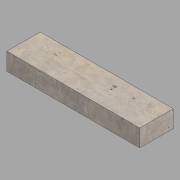
# Autodesk Inventor part: Paver type 2-pedestrian
Saved by Autodesk Inventor 2022 (Build 260153000, 153)
## iProperties
Created: 2021-10-21
Part Number: Paver type 2-pedestrian
Material: Limestone
Document SubType Name: Modeling
Designer: awelt
Density: 2.6 g/cm^3
Appearance: Kasota Gray
Mass: 19098 g
Surface Area: 3056.7 cm^2
Volume: 7345.37 cm^3
Author: awelt
Autodesk Inventor part; units mm, degrees
ref_plane "YZ Plane" through (0, 0, 0) normal (1, 0, 0) x (0, 1, 0)
ref_plane "XZ Plane" through (0, 0, 0) normal (0, 1, 0) x (-1, 0, 0)
ref_plane "XY Plane" through (0, 0, 0) normal (0, 0, 1) x (1, 0, 0)
sketch "Sketch1" plane through (0, 0, 0) normal (0, 1, 0) x (-1, 0, 0)
  line L0 (303.6094, -76.2) -> (-303.6094, -76.2)
  line L1 (-303.6094, -76.2) -> (-303.6094, 76.2)
  line L2 (-303.6094, 76.2) -> (303.6094, 76.2)
  line L3 (303.6094, 76.2) -> (303.6094, -76.2)
  line L4 (303.6094, -76.2) -> (-303.6094, 76.2) construction
  line L5 (-303.6094, -76.2) -> (303.6094, 76.2) construction
  point P0 (0, 0)
  dimension "d0" = 607.2188
  dimension "d1" = 152.4
  constraints: 12 end point, 2 midpoint, 2 parallel, 1 horizontal, 1 perpendicular
  measures "d0" distance of L1.end L2.end
  measures "d1" distance of L0.end L1.end
extrude "Extrusion1" add sketch "Sketch1" along normal blind 79.375
